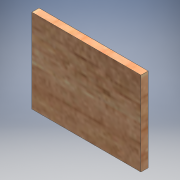
# Autodesk Inventor part: FrontSupportCover
Saved by Autodesk Inventor 2016 (Build 200138000, 138)
## iProperties
Created: 2016-04-01
Part Number: FrontSupportCover
Material: Wood (Birch)
Document SubType Name: Modeling
Designer: mkepler
Mass: 2.62763 g
Surface Area: 36.68 cm^2
Volume: 4.7775 cm^3
Density: 0.55 g/cm^3
Appearance: Birch - Natural Polished
Author: mkepler
Autodesk Inventor part; units mm, degrees
ref_plane "YZ Plane" through (0, 0, 0) normal (1, 0, 0) x (0, 1, 0)
ref_plane "XZ Plane" through (0, 0, 0) normal (0, 1, 0) x (-1, 0, 0)
ref_plane "XY Plane" through (0, 0, 0) normal (0, 0, 1) x (1, 0, 0)
sketch "Sketch1" plane through (0, 0, 0) normal (0, 1, 0) x (-1, 0, 0)
  line L0 (0, 0) -> (45.5, 0)
  line L1 (45.5, 0) -> (45.5, -35)
  line L2 (45.5, -35) -> (0, -35)
  line L3 (0, -35) -> (0, 0)
  dimension "d0" = 45.5
  dimension "d1" = 35
  constraints: 8 end point, 2 parallel, 1 horizontal, 1 perpendicular
  measures "d0" distance of L1.end L2.end
  measures "d1" distance of L0.end L1.end
extrude "Extrusion1" add sketch "Sketch1" along normal blind 3
sketch "Sketch2" plane through (0, 0, -35) normal (0, 0, -1) x (-1, 0, 0)
  circle A0 centre (6, 1.5) radius 1
  line L0 (0, 0) -> (0, 3) projected
  line L1 (45.5, 0) -> (0, 0) projected
  line L2 (0, 0) -> (45.5, 0) projected
  line L3 (22.75, 0) -> (22.75, 1.5)
  circle A1 centre (39.5, 1.5) radius 1
  dimension "d4" = 2
  dimension "d5" = 6
  dimension "d6" = 1.5
  constraints: 2 centre point, 2 end point, 1 midpoint, 1 symmetric about line, 1 vertical, 1 other
  measures "d4" diameter of A0
  measures "d5" distance from line of L0 A0.centre
  measures "d6" distance from line of L1 A0.centre
hole "Hole1" at (-39.5, 1.5, -35) at (-6, 1.5, -35) direction (0, 0, 1) diameter 2 depth 8 tip angle 118
body "Solid1"
